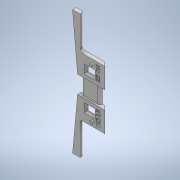
# Autodesk Inventor part: soporte_bat_rachx
Saved by Autodesk Inventor 2020 (Build 240168000, 168)
## iProperties
Created: 2019-03-21
Part Number: soporte_bat_rachx
Material: Genérico
Document SubType Name: Modeling
Designer: UCENTRAL
Density: 1 g/cm^3
Appearance: Valor por defecto
Author: UCENTRAL
Autodesk Inventor part; units mm, degrees
ref_plane "YZ Plane" through (0, 0, 0) normal (1, 0, 0) x (0, 1, 0)
ref_plane "XZ Plane" through (0, 0, 0) normal (0, 1, 0) x (-1, 0, 0)
ref_plane "XY Plane" through (0, 0, 0) normal (0, 0, 1) x (1, 0, 0)
sketch "Boceto2" plane through (0, 0, 0) normal (0, 1, 0) x (-1, 0, 0)
  line L0 (20, 23.5) -> (0, 23.5)
  line L1 (0, 23.5) -> (0, -23.5)
  line L2 (0, -23.5) -> (20, -23.5)
  line L3 (20, -23.5) -> (20, 23.5)
  point P0 (0, 0)
  dimension "d0" = 47
  dimension "d1" = 20
  dimension "d11" = 23.5
  constraints: 8 end point, 2 parallel, 1 horizontal, 1 perpendicular
  measures "d0" distance between parallel lines of L2 L0
  measures "d1" distance between parallel lines of L1 L3
  measures "d11" distance from line of point (0, 0) L0
sketch "Boceto3" plane through (0, 0, 0) normal (0, 1, 0) x (-1, 0, 0)
  line L0 (22, 50) -> (20, 50)
  line L1 (20, 50) -> (20, -50)
  line L2 (20, -50) -> (22, -50)
  line L3 (22, -50) -> (22, 50)
  line L4 (22, 50) -> (26, 50)
  line L5 (26, 50) -> (22, 10.2005)
  line L6 (22, 10.2005) -> (22, 50)
  line L7 (22, -50) -> (26, -50)
  line L8 (26, -50) -> (22, -10.2005)
  line L9 (22, -10.2005) -> (22, -50)
  point P0 (0, 0)
  dimension "d2" = 100
  dimension "d3" = 20
  dimension "d4" = 2
  dimension "d5" = 50
  dimension "d52" = 4
  dimension "d53" = 40
  dimension "d54" = 4
  dimension "d55" = 40
  constraints: 20 end point, 3 horizontal, 3 parallel, 2 point on line, 1 collinear, 1 perpendicular
  measures "d2" distance between parallel lines of L2 L0
  measures "d3" distance from line of point (0, 0) L1
  measures "d4" distance between parallel lines of L3 L1
  measures "d5" distance from line of point (0, 0) L0
  measures "d52" distance of L0.start L4.end
  measures "d53" distance of L4.end L5.end
  measures "d54" distance of L2.end L7.end
  measures "d55" distance of L7.end L8.end
sketch "Boceto5" plane through (0, 0, 0) normal (0, 1, 0) x (-1, 0, 0)
  circle A0 centre (10, 20) radius 1.35
  circle A1 centre (10, -20) radius 1.35
  point P0 (0, 0)
  dimension "d6" = 2.7
  dimension "d7" = 2.7
  dimension "d8" = 40
  dimension "d9" = 10
  dimension "d10" = 20
  dimension "d18" = 10
  constraints: 2 centre point
  measures "d6" diameter of A0
  measures "d7" diameter of A1
  measures "d8" distance of A1.centre A0.centre
  measures "d9" horizontal distance of point (0, 0) A0.centre
  measures "d10" vertical distance of point (0, 0) A0.centre
  measures "d18" horizontal distance of point (0, 0) A1.centre
extrude "Extrusión1" add sketch "Boceto2" along normal blind 3
extrude "Extrusión2" add sketch "Boceto3" along normal blind 3 contours L3 L2 L1 L0
extrude "Extrusión3" add sketch "Boceto5" against normal blind 1
sketch "Boceto7" plane through (0, 3, 0) normal (0, 1, 0) x (1, 0, 0)
  line L0 (-22.0046, -7) -> (-20, -7)
  line L1 (-20, -7) -> (-20, 7)
  line L2 (-20, 7) -> (-22.0046, 7)
  line L3 (-22.0046, 7) -> (-22.0046, -7)
  line L4 (-22, 50) -> (-22, -50) projected
  point P0 (0, 0)
  dimension "d19" = 2
  dimension "d20" = 14
  dimension "d21" = 7
  constraints: 8 end point, 2 parallel, 1 horizontal, 1 perpendicular
  measures "d19" distance between parallel lines of L4 L1
  measures "d20" distance from line of L0.start L2
  measures "d21" distance from line of L0 point (0, 0)
extrude "Extrusión4" cut sketch "Boceto7" against normal blind 3
sketch "Boceto8" plane through (0, 0, 23.5) normal (1, 0, 0) x (0, 0, -1)
  line L0 (30.5, 0) -> (16.5, 0)
  line L1 (16.5, 0) -> (16.5, 1.1)
  line L2 (16.5, 1.1) -> (30.5, 1.1)
  line L3 (30.5, 1.1) -> (30.5, 0)
  point P0 (23.5, 0)
  dimension "d24" = 7
  dimension "d25" = 14
  dimension "d26" = 1.1
  constraints: 8 end point, 2 parallel, 1 horizontal, 1 perpendicular
  measures "d24" distance from line of point (23.5, 0) L3
  measures "d25" distance between parallel lines of L1 L3
  measures "d26" distance between parallel lines of L2 L0
extrude "Extrusión5" cut sketch "Boceto8" against normal blind 50
fillet "Empalme1" radius 2 2 edges at (-20, 1.5, -23.5) (-20, 3, -36.75)
sketch "Boceto9" plane through (0, 1.1, -7) normal (0, -1, 0) x (1, 0, 0)
  line L0 (-22, 14) -> (0, 14) projected
  line L1 (0, 0) -> (-22, 0) projected
  line L2 (0, 14) -> (-5, 14)
  line L3 (-5, 14) -> (-5, 0)
  line L4 (-5, 0) -> (0, 0)
  line L5 (0, 0) -> (0, 14)
  point P0 (0, 7)
  dimension "d31" = 5
  constraints: 8 end point, 2 parallel, 1 horizontal, 1 perpendicular, 1 point on line
  measures "d31" distance between parallel lines of L3 L5
extrude "Extrusión6" cut sketch "Boceto9" against normal blind 50
fillet "Empalme3" radius 2 1 edges at (-20, 3, 36.75)
fillet "Empalme4" radius 2 2 edges at (-20.5858, 2.4142, 23.5) (-20, 0.5001, 23.5)
chamfer "Chaflán1" distance 3 angle 45 1 edges at (0, 3, -15.25)
chamfer "Chaflán2" distance 3 angle 45 1 edges at (0, 3, 15.25)
fillet "Empalme5" radius 2 1 edges at (-5, 1.1, 0)
fillet "Empalme6" radius 2 1 edges at (-20, 1.1, 0)
sketch "Boceto10" plane through (0, 3, 0) normal (0, 1, 0) x (1, 0, 0)
  line L0 (-7.1179, -21.5947) -> (-7.1179, -10.7865) construction
  line L1 (-7.1179, -10.7865) -> (-3.9612, -10.7865) construction
  line L2 (-3.9612, -10.7865) -> (-3.9612, -21.5947) construction
  line L3 (-3.9612, -21.5947) -> (-7.1179, -21.5947) construction
  line L4 (-7.1296, 9.1761) -> (-7.1296, 23.1861) construction
  line L5 (-7.1296, 23.1861) -> (-3.9531, 23.1861) construction
  line L6 (-3.9531, 23.1861) -> (-3.9531, 9.1761) construction
  line L7 (-3.9531, 9.1761) -> (-7.1296, 9.1761) construction
  line L8 (-4.0056, -19.1049) -> (-4.0056, -19.5594)
  line L9 (-4.0056, -19.5594) -> (-6.6337, -20.908)
  line L10 (-6.6337, -20.908) -> (-4.0056, -20.908)
  line L11 (-4.0056, -20.908) -> (-4.0056, -21.2859)
  line L12 (-4.0056, -21.2859) -> (-7.0536, -21.2859)
  line L13 (-7.0536, -21.2859) -> (-7.0536, -20.7104)
  line L14 (-7.0536, -20.7104) -> (-4.6404, -19.4828)
  line L15 (-4.6404, -19.4828) -> (-7.0536, -19.4828)
  line L16 (-7.0536, -19.4828) -> (-7.0536, -19.1049)
  line L17 (-7.0536, -19.1049) -> (-4.0056, -19.1049)
  spline S0 degree 2 poles (-6.7054, -16.331) (-6.5028, -16.1581) (-5.91, -15.9655) (-5.5296, -15.9655) knots 0 0 0 1 2 2 2
  spline S1 degree 2 poles (-5.5296, -15.9655) (-5.1591, -15.9655) (-4.5589, -16.1532) (-4.3564, -16.331) knots 0 0 0 1 2 2 2
  spline S2 degree 2 poles (-4.3564, -16.331) (-4.144, -16.5188) (-3.9414, -17.0152) (-3.9414, -17.3141) knots 0 0 0 1 2 2 2
  spline S3 degree 2 poles (-3.9414, -17.3141) (-3.9414, -17.6229) (-4.1514, -18.1169) (-4.3564, -18.2972) knots 0 0 0 1 2 2 2
  spline S4 degree 2 poles (-4.3564, -18.2972) (-4.5589, -18.4726) (-5.1542, -18.6603) (-5.5296, -18.6603) knots 0 0 0 1 2 2 2
  spline S5 degree 2 poles (-5.5296, -18.6603) (-5.9125, -18.6603) (-6.4954, -18.4701) (-6.7054, -18.2947) knots 0 0 0 1 2 2 2
  spline S6 degree 2 poles (-6.7054, -18.2947) (-6.9079, -18.1169) (-7.1179, -17.6204) (-7.1179, -17.3141) knots 0 0 0 1 2 2 2
  spline S7 degree 2 poles (-7.1179, -17.3141) (-7.1179, -17.0029) (-6.9005, -16.5039) (-6.7054, -16.331) knots 0 0 0 1 2 2 2
  spline S8 degree 2 poles (-5.5296, -16.3879) (-5.831, -16.3879) (-6.2978, -16.5188) (-6.451, -16.6373) knots 0 0 0 1 2 2 2
  spline S9 degree 2 poles (-6.451, -16.6373) (-6.609, -16.7584) (-6.7671, -17.0992) (-6.7671, -17.3116) knots 0 0 0 1 2 2 2
  spline S10 degree 2 poles (-6.7671, -17.3116) (-6.7671, -17.5315) (-6.614, -17.8625) (-6.451, -17.9884) knots 0 0 0 1 2 2 2
  spline S11 degree 2 poles (-6.451, -17.9884) (-6.2953, -18.1095) (-5.826, -18.2379) (-5.5296, -18.2379) knots 0 0 0 1 2 2 2
  spline S12 degree 2 poles (-5.5296, -18.2379) (-4.9294, -18.2379) (-4.2922, -17.734) (-4.2922, -17.3116) knots 0 0 0 1 2 2 2
  spline S13 degree 2 poles (-4.2922, -17.3116) (-4.2922, -16.8893) (-4.9294, -16.3879) (-5.5296, -16.3879) knots 0 0 0 1 2 2 2
  line L18 (-4.0056, -14.2118) -> (-7.0536, -14.2118)
  line L19 (-7.0536, -14.2118) -> (-7.0536, -12.3049)
  line L20 (-7.0536, -12.3049) -> (-6.693, -12.3049)
  line L21 (-6.693, -12.3049) -> (-6.693, -13.8067)
  line L22 (-6.693, -13.8067) -> (-5.8582, -13.8067)
  line L23 (-5.8582, -13.8067) -> (-5.8582, -12.4062)
  line L24 (-5.8582, -12.4062) -> (-5.4975, -12.4062)
  line L25 (-5.4975, -12.4062) -> (-5.4975, -13.8067)
  line L26 (-5.4975, -13.8067) -> (-4.3663, -13.8067)
  line L27 (-4.3663, -13.8067) -> (-4.3663, -12.3049)
  line L28 (-4.3663, -12.3049) -> (-4.0056, -12.3049)
  line L29 (-4.0056, -12.3049) -> (-4.0056, -14.2118)
  spline S14 degree 2 poles (-3.9513, -11.0106) (-3.9513, -11.3416) (-4.0896, -11.806) (-4.1884, -12.011) knots 0 0 0 1 2 2 2
  line L30 (-4.1884, -12.011) -> (-4.6972, -12.011)
  line L31 (-4.6972, -12.011) -> (-4.6972, -11.9813)
  spline S15 degree 2 poles (-4.6972, -11.9813) (-4.5095, -11.7813) (-4.302, -11.2749) (-4.302, -11.0403) knots 0 0 0 1 2 2 2
  spline S16 degree 2 poles (-4.302, -11.0403) (-4.302, -10.7043) (-4.5812, -10.361) (-4.8109, -10.361) knots 0 0 0 1 2 2 2
  spline S17 degree 2 poles (-4.8109, -10.361) (-4.9936, -10.361) (-5.2209, -10.5413) (-5.2777, -10.7365) knots 0 0 0 1 2 2 2
  spline S18 degree 2 poles (-5.2777, -10.7365) (-5.3172, -10.8773) (-5.3716, -11.1119) (-5.416, -11.2873) knots 0 0 0 1 2 2 2
  spline S19 degree 2 poles (-5.416, -11.2873) (-5.458, -11.4454) (-5.584, -11.6948) (-5.6852, -11.7912) knots 0 0 0 1 2 2 2
  spline S20 degree 2 poles (-5.6852, -11.7912) (-5.7865, -11.885) (-6.0582, -11.9888) (-6.2361, -11.9888) knots 0 0 0 1 2 2 2
  spline S21 degree 2 poles (-6.2361, -11.9888) (-6.6066, -11.9888) (-7.108, -11.4108) (-7.108, -10.9637) knots 0 0 0 1 2 2 2
  spline S22 degree 2 poles (-7.108, -10.9637) (-7.108, -10.7068) (-7.0067, -10.2523) (-6.9104, -10.0572) knots 0 0 0 1 2 2 2
  line L32 (-6.9104, -10.0572) -> (-6.4263, -10.0572)
  line L33 (-6.4263, -10.0572) -> (-6.4263, -10.0868)
  spline S23 degree 2 poles (-6.4263, -10.0868) (-6.5596, -10.2326) (-6.7572, -10.6871) (-6.7572, -10.9365) knots 0 0 0 1 2 2 2
  spline S24 degree 2 poles (-6.7572, -10.9365) (-6.7572, -11.2181) (-6.4929, -11.5664) (-6.2781, -11.5664) knots 0 0 0 1 2 2 2
  spline S25 degree 2 poles (-6.2781, -11.5664) (-6.0854, -11.5664) (-5.8557, -11.3614) (-5.8038, -11.1687) knots 0 0 0 1 2 2 2
  spline S26 degree 2 poles (-5.8038, -11.1687) (-5.7692, -11.0403) (-5.6803, -10.6673) (-5.6433, -10.5438) knots 0 0 0 1 2 2 2
  spline S27 degree 2 poles (-5.6433, -10.5438) (-5.5469, -10.2301) (-5.1591, -9.9386) (-4.8751, -9.9386) knots 0 0 0 1 2 2 2
  spline S28 degree 2 poles (-4.8751, -9.9386) (-4.6948, -9.9386) (-4.349, -10.0844) (-4.2279, -10.2153) knots 0 0 0 1 2 2 2
  spline S29 degree 2 poles (-4.2279, -10.2153) (-4.0946, -10.361) (-3.9513, -10.7315) (-3.9513, -11.0106) knots 0 0 0 1 2 2 2
  line L34 (-3.8673, 12.4643) -> (-3.8673, 11.4867)
  line L35 (-3.8673, 11.4867) -> (-5.0421, 10.5972)
  line L36 (-5.0421, 10.5972) -> (-5.0421, 10.3068)
  line L37 (-5.0421, 10.3068) -> (-3.8673, 10.3068)
  line L38 (-3.8673, 10.3068) -> (-3.8673, 9.5081)
  line L39 (-3.8673, 9.5081) -> (-7.0673, 9.5081)
  line L40 (-7.0673, 9.5081) -> (-7.0673, 10.7943)
  spline S30 degree 2 poles (-7.0673, 10.7943) (-7.0673, 11.0614) (-6.9999, 11.4555) (-6.8962, 11.6241) knots 0 0 0 1 2 2 2
  spline S31 degree 2 poles (-6.8962, 11.6241) (-6.7873, 11.7953) (-6.4476, 11.9975) (-6.1883, 11.9975) knots 0 0 0 1 2 2 2
  spline S32 degree 2 poles (-6.1883, 11.9975) (-5.8226, 11.9975) (-5.3636, 11.6656) (-5.2288, 11.3881) knots 0 0 0 1 2 2 2
  line L41 (-5.2288, 11.3881) -> (-3.8673, 12.4643)
  spline S33 degree 2 poles (-6.0871, 11.1729) (-6.209, 11.1729) (-6.3827, 11.0795) (-6.4294, 10.9732) knots 0 0 0 1 2 2 2
  spline S34 degree 2 poles (-6.4294, 10.9732) (-6.4605, 10.898) (-6.4787, 10.7139) (-6.4787, 10.5765) knots 0 0 0 1 2 2 2
  line L42 (-6.4787, 10.5765) -> (-6.4787, 10.3068)
  line L43 (-6.4787, 10.3068) -> (-5.6178, 10.3068)
  line L44 (-5.6178, 10.3068) -> (-5.6178, 10.5376)
  spline S35 degree 2 poles (-5.6178, 10.5376) (-5.6178, 10.7035) (-5.6592, 10.9395) (-5.7241, 11.0199) knots 0 0 0 1 2 2 2
  spline S36 degree 2 poles (-5.7241, 11.0199) (-5.7863, 11.0977) (-5.9523, 11.1729) (-6.0871, 11.1729) knots 0 0 0 1 2 2 2
  line L45 (-3.8673, 12.358) -> (-7.0673, 13.4393)
  line L46 (-7.0673, 13.4393) -> (-7.0673, 14.3158)
  line L47 (-7.0673, 14.3158) -> (-3.8673, 15.3972)
  line L48 (-3.8673, 15.3972) -> (-3.8673, 14.57)
  line L49 (-3.8673, 14.57) -> (-4.5208, 14.3703)
  line L50 (-4.5208, 14.3703) -> (-4.5208, 13.3641)
  line L51 (-4.5208, 13.3641) -> (-3.8673, 13.1619)
  line L52 (-3.8673, 13.1619) -> (-3.8673, 12.358)
  line L53 (-5.1017, 14.194) -> (-6.1597, 13.8672)
  line L54 (-6.1597, 13.8672) -> (-5.1017, 13.5379)
  line L55 (-5.1017, 13.5379) -> (-5.1017, 14.194)
  spline S37 degree 2 poles (-3.8051, 17.0957) (-3.8051, 16.3748) (-4.6764, 15.5295) (-5.4648, 15.5295) knots 0 0 0 1 2 2 2
  spline S38 degree 2 poles (-5.4648, 15.5295) (-6.2246, 15.5295) (-7.1296, 16.3774) (-7.1296, 17.0983) knots 0 0 0 1 2 2 2
  spline S39 degree 2 poles (-7.1296, 17.0983) (-7.1296, 17.2876) (-7.0855, 17.5936) (-7.0492, 17.7337) knots 0 0 0 1 2 2 2
  spline S40 degree 2 poles (-7.0492, 17.7337) (-7.0155, 17.8426) (-6.904, 18.0993) (-6.8625, 18.1797) knots 0 0 0 1 2 2 2
  line L56 (-6.8625, 18.1797) -> (-6.1001, 18.1797)
  line L57 (-6.1001, 18.1797) -> (-6.1001, 18.0993)
  spline S41 degree 2 poles (-6.1001, 18.0993) (-6.1519, 18.0397) (-6.2972, 17.8633) (-6.3646, 17.7518) knots 0 0 0 1 2 2 2
  spline S42 degree 2 poles (-6.3646, 17.7518) (-6.4346, 17.6403) (-6.5306, 17.3732) (-6.5306, 17.2254) knots 0 0 0 1 2 2 2
  spline S43 degree 2 poles (-6.5306, 17.2254) (-6.5306, 17.0517) (-6.4216, 16.7638) (-6.2842, 16.6316) knots 0 0 0 1 2 2 2
  spline S44 degree 2 poles (-6.2842, 16.6316) (-6.1623, 16.5123) (-5.7448, 16.3593) (-5.4622, 16.3593) knots 0 0 0 1 2 2 2
  spline S45 degree 2 poles (-5.4622, 16.3593) (-5.1639, 16.3593) (-4.7568, 16.5175) (-4.6323, 16.6471) knots 0 0 0 1 2 2 2
  spline S46 degree 2 poles (-4.6323, 16.6471) (-4.5105, 16.7716) (-4.4041, 17.0776) (-4.4041, 17.2306) knots 0 0 0 1 2 2 2
  spline S47 degree 2 poles (-4.4041, 17.2306) (-4.4041, 17.3888) (-4.5105, 17.6766) (-4.5753, 17.7752) knots 0 0 0 1 2 2 2
  spline S48 degree 2 poles (-4.5753, 17.7752) (-4.6401, 17.8841) (-4.7776, 18.0474) (-4.832, 18.1071) knots 0 0 0 1 2 2 2
  line L58 (-4.832, 18.1071) -> (-4.832, 18.1797)
  line L59 (-4.832, 18.1797) -> (-4.08, 18.1797)
  spline S49 degree 2 poles (-4.08, 18.1797) (-4.0385, 18.0915) (-3.9348, 17.8607) (-3.8985, 17.7363) knots 0 0 0 1 2 2 2
  spline S50 degree 2 poles (-3.8985, 17.7363) (-3.8518, 17.5859) (-3.8051, 17.3239) (-3.8051, 17.0957) knots 0 0 0 1 2 2 2
  line L60 (-3.8673, 21.3538) -> (-3.8673, 20.5499)
  line L61 (-3.8673, 20.5499) -> (-5.2858, 20.5499)
  line L62 (-5.2858, 20.5499) -> (-5.2858, 19.4581)
  line L63 (-5.2858, 19.4581) -> (-3.8673, 19.4581)
  line L64 (-3.8673, 19.4581) -> (-3.8673, 18.6543)
  line L65 (-3.8673, 18.6543) -> (-7.0673, 18.6543)
  line L66 (-7.0673, 18.6543) -> (-7.0673, 19.4581)
  line L67 (-7.0673, 19.4581) -> (-5.8952, 19.4581)
  line L68 (-5.8952, 19.4581) -> (-5.8952, 20.5499)
  line L69 (-5.8952, 20.5499) -> (-7.0673, 20.5499)
  line L70 (-7.0673, 20.5499) -> (-7.0673, 21.3538)
  line L71 (-7.0673, 21.3538) -> (-3.8673, 21.3538)
  point P0 (0, 0)
  constraints: 4 other
extrude "Extrusión7" cut sketch "Boceto10" against normal blind 50
sketch "Boceto12" plane through (0, 0, 0) normal (0, -1, 0) x (1, 0, 0)
  line L0 (-7.8329, 17) -> (-16.5484, 17)
  line L1 (-16.5484, 17) -> (-16.5484, 10)
  line L2 (-16.5484, 10) -> (-7.8329, 10)
  line L3 (-7.8329, 10) -> (-7.8329, 17)
  line L4 (-16.5484, -10) -> (-7.8329, -10)
  line L5 (-7.8329, -10) -> (-7.8329, -17)
  line L6 (-7.8329, -17) -> (-16.5484, -17)
  line L7 (-16.5484, -17) -> (-16.5484, -10)
  point P0 (0, 0)
  dimension "d46" = 7
  dimension "d47" = 10
  dimension "d48" = 10
  dimension "d49" = 7
  constraints: 16 end point, 4 parallel, 2 horizontal, 2 perpendicular, 2 point on line
  measures "d46" distance between parallel lines of L2 L0
  measures "d47" distance from line of point (0, 0) L2
  measures "d48" distance from line of point (0, 0) L4
  measures "d49" distance between parallel lines of L4 L6
extrude "Extrusión8" cut sketch "Boceto12" against normal blind 50
sketch "Boceto14" plane through (0, 0, 0) normal (0, -1, 0) x (1, 0, 0)
  line L0 (-22, 50) -> (-20, 50) projected
  line L1 (-22, 50) -> (-26, 50)
  line L2 (-22, 7) -> (-22, 25.5) projected
  line L3 (-26, 50) -> (-22, 7)
  line L4 (-22, 7) -> (-22, 50)
  line L5 (-22, -7) -> (-20, -7) projected
  line L6 (-22, -50) -> (-22, -7) projected
  line L7 (-22, -7) -> (-22, -50)
  line L8 (-22, -50) -> (-26, -50)
  line L9 (-26, -50) -> (-22, -7)
  point P0 (0, 0)
  dimension "d56" = 4
  dimension "d57" = 4
  constraints: 12 end point, 1 collinear, 1 horizontal, 1 perpendicular, 1 vertical
  measures "d56" distance of L0.start L1.end
  measures "d57" distance of L6.start L8.end
extrude "Extrusión9" add sketch "Boceto14" against normal blind 3
